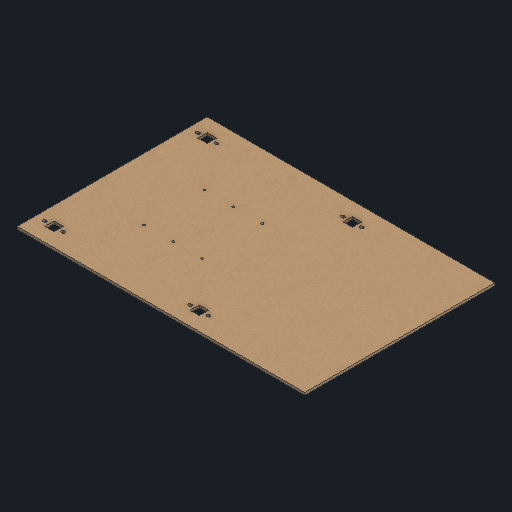
# Autodesk Inventor part: UpperBase
Saved by Autodesk Inventor 2027.1 (Build 311270010, 270A)
## iProperties
Created: 2026-09-29
Part Number: UpperBase
Material: MDF Medium Density Fiberboard
Document SubType Name: Modeling
Designer: SDS Scholar
Density: 0.8 g/cm^3
Appearance: Cardboard - Corrugated
Author: SDS Scholar
Autodesk Inventor part; units mm, degrees
ref_plane "YZ Plane" through (0, 0, 0) normal (1, 0, 0) x (0, 1, 0)
ref_plane "XZ Plane" through (0, 0, 0) normal (0, 1, 0) x (-1, 0, 0)
ref_plane "XY Plane" through (0, 0, 0) normal (0, 0, 1) x (1, 0, 0)
sketch "Sketch1" plane through (0, 0, 0) normal (0, 1, 0) x (-1, 0, 0)
  line L0 (312, 206) -> (-312, 206)
  line L1 (-312, 206) -> (-312, -206)
  line L2 (-312, -206) -> (312, -206)
  line L3 (312, -206) -> (312, 206)
  circle A0 centre (177.5, 65.5) radius 2.5
  line L4 (0, 206) -> (0, -206) construction
  line L5 (312, 0) -> (-312, 0) construction
  circle A1 centre (177.5, -65.5) radius 2.5
  circle A2 centre (114.5, 65.5) radius 2.5
  circle A3 centre (114.5, -65.5) radius 2.5
  circle A4 centre (51.5, 65.5) radius 2.5
  circle A5 centre (51.5, -65.5) radius 2.5
  line L6 (282, -176) -> (262, -176)
  line L7 (262, -176) -> (262, -156)
  line L8 (262, -156) -> (282, -156)
  line L9 (282, -156) -> (282, -176)
  line L10 (-83, -206) -> (-83, 206)
  line L11 (253.5, -166) -> (250.5, -166) construction
  line L12 (253.5, -163.1) -> (250.5, -163.1)
  line L13 (250.5, -168.9) -> (253.5, -168.9)
  arc A6 (253.5, -168.9) -> (253.5, -163.1) centre (253.5, -166) ccw
  arc A7 (250.5, -163.1) -> (250.5, -168.9) centre (250.5, -166) ccw
  line L14 (272, -176) -> (272, -156) construction
  line L15 (290.5, -166) -> (293.5, -166) construction
  line L16 (290.5, -163.1) -> (293.5, -163.1)
  line L17 (293.5, -168.9) -> (290.5, -168.9)
  arc A8 (290.5, -163.1) -> (290.5, -168.9) centre (290.5, -166) ccw
  arc A9 (293.5, -168.9) -> (293.5, -163.1) centre (293.5, -166) ccw
  line L18 (282, -166) -> (262, -166) construction
  line L19 (114.5, 206) -> (114.5, -206) construction
  arc A10 (250.5, 168.9) -> (250.5, 163.1) centre (250.5, 166) ccw
  line L20 (282, 176) -> (282, 156)
  arc A11 (290.5, 168.9) -> (290.5, 163.1) centre (290.5, 166) ccw
  line L21 (290.5, 166) -> (293.5, 166) construction
  line L22 (293.5, 163.1) -> (290.5, 163.1)
  arc A12 (293.5, 163.1) -> (293.5, 168.9) centre (293.5, 166) ccw
  line L23 (290.5, 168.9) -> (293.5, 168.9)
  line L24 (282, 156) -> (262, 156)
  line L25 (272, 156) -> (272, 176) construction
  line L26 (282, 166) -> (262, 166) construction
  line L27 (262, 176) -> (282, 176)
  line L28 (262, 156) -> (262, 176)
  arc A13 (253.5, 163.1) -> (253.5, 168.9) centre (253.5, 166) ccw
  line L29 (253.5, 168.9) -> (250.5, 168.9)
  line L30 (253.5, 166) -> (250.5, 166) construction
  line L31 (250.5, 163.1) -> (253.5, 163.1)
  arc A14 (-64.5, -163.1) -> (-64.5, -168.9) centre (-64.5, -166) ccw
  line L32 (-33, -156) -> (-33, -176)
  arc A15 (-24.5, -163.1) -> (-24.5, -168.9) centre (-24.5, -166) ccw
  line L33 (-24.5, -166) -> (-21.5, -166) construction
  line L34 (-21.5, -168.9) -> (-24.5, -168.9)
  arc A16 (-21.5, -168.9) -> (-21.5, -163.1) centre (-21.5, -166) ccw
  line L35 (-24.5, -163.1) -> (-21.5, -163.1)
  line L36 (-33, -176) -> (-53, -176)
  line L37 (-43, -176) -> (-43, -156) construction
  line L38 (-33, -166) -> (-53, -166) construction
  line L39 (-53, -156) -> (-33, -156)
  line L40 (-53, -176) -> (-53, -156)
  arc A17 (-61.5, -168.9) -> (-61.5, -163.1) centre (-61.5, -166) ccw
  line L41 (-61.5, -163.1) -> (-64.5, -163.1)
  line L42 (-61.5, -166) -> (-64.5, -166) construction
  line L43 (-64.5, -168.9) -> (-61.5, -168.9)
  arc A18 (-64.5, 168.9) -> (-64.5, 163.1) centre (-64.5, 166) ccw
  line L44 (-33, 176) -> (-33, 156)
  arc A19 (-24.5, 168.9) -> (-24.5, 163.1) centre (-24.5, 166) ccw
  line L45 (-24.5, 166) -> (-21.5, 166) construction
  line L46 (-21.5, 163.1) -> (-24.5, 163.1)
  arc A20 (-21.5, 163.1) -> (-21.5, 168.9) centre (-21.5, 166) ccw
  line L47 (-24.5, 168.9) -> (-21.5, 168.9)
  line L48 (-33, 156) -> (-53, 156)
  line L49 (-43, 156) -> (-43, 176) construction
  line L50 (-33, 166) -> (-53, 166) construction
  line L51 (-53, 176) -> (-33, 176)
  line L52 (-53, 156) -> (-53, 176)
  arc A21 (-61.5, 163.1) -> (-61.5, 168.9) centre (-61.5, 166) ccw
  line L53 (-61.5, 168.9) -> (-64.5, 168.9)
  line L54 (-61.5, 166) -> (-64.5, 166) construction
  line L55 (-64.5, 163.1) -> (-61.5, 163.1)
  point P0 (0, 0)
  point P1 (-83, 0)
  point P2 (252, -166)
  point P3 (292, -166)
  point P4 (272, -166)
  point P5 (114.5, 0)
  point P6 (292, 166)
  point P7 (272, 166)
  point P8 (252, 166)
  point P9 (-23, -166)
  point P10 (-43, -166)
  point P11 (-63, -166)
  point P12 (-23, 166)
  point P13 (-43, 166)
  point P14 (-63, 166)
  dimension "d0" = 412
  dimension "d1" = 624
  dimension "d3" = 5
  dimension "d6" = 131
  dimension "d9" = 63
  dimension "d15" = 20
  dimension "d16" = 20
  dimension "d17" = 30
  dimension "d18" = 30
  dimension "d26" = 1.5
  dimension "d27" = 5.8
  dimension "d28" = 8.5
  dimension "d51" = 395
  dimension "d52" = 197.5
  dimension "d63" = 332
  dimension "d66" = 315
  constraints: 128 end point, 32 point on circle, 22 centre point, 12 midpoint, 7 symmetric about line, 5 horizontal, 5 parallel, 5 perpendicular, 4 point on line, 4 tangent, 3 vertical, 2 horizontal alignment, 2 vertical alignment, 130 other
  measures "d0" distance of L2.end L0.start
  measures "d1" distance of L1.end L2.end
  measures "d3" diameter of A0
  measures "d6" distance of A0.centre A1.centre
  measures "d9" distance of A0.centre A2.centre
  measures "d15" distance of L7.end L8.end
  measures "d16" distance of L6.end L7.end
  measures "d17" distance between parallel lines of L2 L6
  measures "d18" distance between parallel lines of L3 L9
  measures "d26" distance of point (252, -166) L11.end
  measures "d27" diameter of A7
  measures "d28" distance from line of L7 L11.start
  measures "d51" distance between parallel lines of L3 L10
  measures "d52" distance between parallel lines of L3 L19
  measures "d63" distance of L11.end L30.end
  measures "d66" distance of L11.end L42.end
extrude "Extrusion1" add sketch "Sketch1" along normal blind 5 contours L3 L2 L10 L0 | L10 L2 L1 L0 | L6 L7 L8 L9 | A6 L13 A7 L12 | L16 A9 L17 A8 | L29 A13 L31 A10 | L20 L24 L28 L27 | L23 A12 L22 A11 | L41 A17 L43 A14 | L32 L36 L40 L39 | L35 A16 L34 A15 | L53 A21 L55 A18 | L44 L48 L52 L51 | L47 A20 L46 A19
extrude "Extrusion2" cut sketch "Sketch1" along normal through all contours L6 L7 L8 L9 | A6 L13 A7 L12 | L16 A9 L17 A8 | L29 A13 L31 A10 | L20 L24 L28 L27 | L23 A12 L22 A11 | L41 A17 L43 A14 | L32 L36 L40 L39 | L35 A16 L34 A15 | L53 A21 L55 A18 | L44 L48 L52 L51 | L47 A20 L46 A19
equation "\"d0\" = BaseTotalWidth"
equation "\"d1\" = BaseTotalLength"
equation "\"d6\" = 2 * GridTotalSize + DistanceBetweenGrid"
equation "\"d9\" = GridTotalSize"
equation "\"d15\" = AluminiumExtrusionBase"
equation "\"d16\" = AluminiumExtrusionBase"
equation "\"d17\" = AluminiumExtrusionClearance"
equation "\"d18\" = AluminiumExtrusionClearance"
equation "\"d51\" = WorkspaceLength"
equation "\"d52\" = 0.5 * WorkspaceLength"
equation "\"d63\" = WorkspaceWidth"
equation "\"d66\" = -2 * AluminiumExtrusionClearance + WorkspaceLength - AluminiumExtrusionBase"
equation "\"GridBorderThickness\" = 5"
equation "\"GridBorderFillets\" = 7"
equation "\"GridTotalSize\" = 63"
equation "\"GridProcutClearance\" = 3"
equation "\"AluminiumExtrusionBase\" = 20"
equation "\"AluminiumExtrusionClearance\" = 30"
equation "\"BaseTotalWidth\" = 412"
equation "\"BaseTotalLength\" = 624"
equation "\"DistanceBetweenGrid\" = 5"
equation "\"WorkspaceLength\" = 395"
equation "\"WorkspaceWidth\" = 332"
equation "\"AxesBaseFillet\" = 15"
equation "\"Zaxis\" = 127"
body "Solid1"
